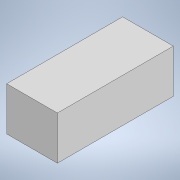
# Autodesk Inventor part: Weapon-Electric-Body
Saved by Autodesk Inventor 2020 (Build 240168000, 168)
## iProperties
Created: 2019-11-14
Part Number: Weapon-Electric-Body
Material: Generic
Document SubType Name: Modeling
Designer: vifly_01
Density: 1 g/cm^3
Appearance: Default
Author: vifly_01
Autodesk Inventor part; units mm, degrees
ref_plane "YZ Plane" through (0, 0, 0) normal (1, 0, 0) x (0, 1, 0)
ref_plane "XZ Plane" through (0, 0, 0) normal (0, 1, 0) x (-1, 0, 0)
ref_plane "XY Plane" through (0, 0, 0) normal (0, 0, 1) x (1, 0, 0)
sketch "Sketch1" plane through (0, 0, 0) normal (0, 0, 1) x (1, 0, 0)
  line L0 (8.75, -7.5) -> (-8.75, -7.5)
  line L1 (-8.75, -7.5) -> (-8.75, 7.5)
  line L2 (-8.75, 7.5) -> (8.75, 7.5)
  line L3 (8.75, 7.5) -> (8.75, -7.5)
  line L4 (8.75, -7.5) -> (-8.75, 7.5) construction
  line L5 (-8.75, -7.5) -> (8.75, 7.5) construction
  point P0 (0, 0)
  dimension "d0" = 17.5
  dimension "d1" = 15
  constraints: 12 end point, 2 midpoint, 2 parallel, 1 horizontal, 1 perpendicular
  measures "d0" distance of L1.end L2.end
  measures "d1" distance of L0.end L1.end
extrude "Extrusion1" add sketch "Sketch1" along normal blind 40
body "Solid1"
